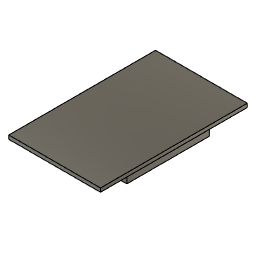
Stack_Up_v2 (Autodesk Fusion 360 archive; units mm, degrees)
design "IO Boards"
Autodesk Fusion 360 part; units mm, degrees
(part 1 of 2)
sketch "Sketch1" plane through (0, 0, 0) normal (0, 0, 1) x (1, 0, 0)
  line L0 (0, 0) -> (40, 0)
  line L1 (40, 0) -> (40, 64)
  line L2 (40, 64) -> (0, 64)
  line L3 (0, 64) -> (0, 0)
  dimension "d1" = 40
  dimension "d2" = 64
  constraint horizontal L0
  constraint vertical L1
  constraint horizontal L2
  constraint vertical L3
  constraint coincident L0.start L3.end
  measures "d1" distance of L0.start L0.end
  measures "d2" distance of L0.start L2.end
extrude "Extrude1" add sketch "Sketch1" along normal blind 1.6
sketch "Sketch4" plane through (0, 0, 0) normal (0, 0, 1) x (1, 0, 0)
  line L0 (0, 0) -> (0, 32) construction
  line L1 (0, 32) -> (40, 32) construction
  line L2 (0, 32) -> (5, 32) construction
  line L3 (40, 32) -> (35, 32) construction
  line L4 (7.5, 50) -> (2.5, 50)
  line L5 (2.5, 50) -> (2.5, 14)
  line L6 (2.5, 14) -> (7.5, 14)
  line L7 (7.5, 14) -> (7.5, 50)
  line L8 (7.5, 50) -> (2.5, 14) construction
  line L9 (2.5, 50) -> (7.5, 14) construction
  line L10 (37.5, 50) -> (32.5, 50)
  line L11 (32.5, 50) -> (32.5, 14)
  line L12 (32.5, 14) -> (37.5, 14)
  line L13 (37.5, 14) -> (37.5, 50)
  line L14 (37.5, 50) -> (32.5, 14) construction
  line L15 (32.5, 50) -> (37.5, 14) construction
  point P0 (5, 32)
  point P1 (35, 32)
  dimension "d23" = 32
  dimension "d24" = 5
  dimension "d25" = 5
  dimension "d26" = 5
  dimension "d27" = 36
  dimension "d28" = 5
  dimension "d29" = 36
  constraint coincident L0.start origin
  constraint vertical L0
  constraint perpendicular L0 L1
  constraint perpendicular L0 L2
  constraint parallel L1 L3
  constraint horizontal L4
  constraint perpendicular L4 L5
  constraint parallel L4 L6
  constraint parallel L5 L7
  constraint coincident L8 P0
  constraint coincident L9 P0
  constraint coincident P0 L2.end
  constraint horizontal L10
  constraint perpendicular L10 L11
  constraint parallel L10 L12
  constraint parallel L11 L13
  constraint coincident L14 P1
  constraint coincident L15 P1
  constraint coincident P1 L3.end
  measures "d23" distance of L0.start L0.end
  measures "d24" distance of L0.end P0
  measures "d25" distance of L1.end P1
  measures "d26" distance of L5.end L6.end
  measures "d27" distance of L4.end L5.end
  measures "d28" distance of L11.end L12.end
  measures "d29" distance of L10.end L11.end
extrude "Extrude6" add sketch "Sketch4" against normal blind 5.08

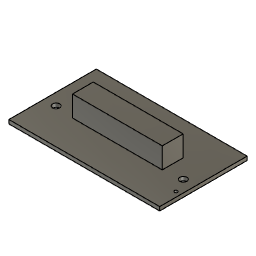
design "Output Board"
Autodesk Fusion 360 part; units mm, degrees
sketch "Sketch1" plane through (0, 0, 0) normal (0, 0, 1) x (1, 0, 0)
  line L0 (0, 0) -> (63.8, 0)
  line L1 (63.8, 0) -> (63.8, 37)
  line L2 (63.8, 37) -> (0, 37)
  line L3 (0, 37) -> (0, 0)
  dimension "d1" = 63.8
  dimension "d2" = 37
  constraint horizontal L0
  constraint vertical L1
  constraint horizontal L2
  constraint vertical L3
  constraint coincident L0.start L3.end
  measures "d1" distance of L0.start L0.end
  measures "d2" distance of L0.start L2.end
extrude "Extrude1" add sketch "Sketch1" along normal blind 1.6
sketch "Sketch2" plane through (0, 0, 1.6) normal (0, 0, 1) x (-1, 0, 0)
  line L0 (0, -37) -> (0, 0)
  line L1 (0, 0) -> (-63.8, 0)
  line L2 (-63.8, 0) -> (-63.8, -37)
  line L3 (-63.8, -37) -> (0, -37)
  line L4 (-50.9, -14) -> (-12.9, -14)
  line L5 (-12.9, -14) -> (-12.9, -22.8)
  line L6 (-12.9, -22.8) -> (-50.9, -22.8)
  line L7 (-50.9, -22.8) -> (-50.9, -14)
  line L8 (-50.9, -14) -> (-12.9, -22.8) construction
  line L9 (-12.9, -14) -> (-50.9, -22.8) construction
  point P0 (-31.9, -18.4)
  dimension "d6" = 38
  dimension "d7" = 8.8
  dimension "d32" = 18.4
  dimension "d33" = 31.9
  constraint horizontal L4
  constraint perpendicular L4 L5
  constraint parallel L4 L6
  constraint parallel L5 L7
  constraint coincident L8 P0
  constraint coincident L9 P0
  measures "d6" distance of L5.end L6.end
  measures "d7" distance of L4.end L5.end
  measures "d32" distance of L1 P0
  measures "d33" distance of L0 P0
extrude "Extrude2" add sketch "Sketch2" along normal blind 8.8 contours L4 L5 L6 L7
sketch "Sketch3" plane through (0, 0, 1.6) normal (0, 0, 1) x (-1, 0, 0)
  line L0 (-50.9, -22.8) -> (-50.9, -14)
  line L1 (-50.9, -14) -> (-12.9, -14)
  line L2 (-12.9, -14) -> (-12.9, -22.8)
  line L3 (-12.9, -22.8) -> (-50.9, -22.8)
  line L4 (0, -37) -> (0, 0)
  line L5 (0, 0) -> (-63.8, 0)
  line L6 (-63.8, 0) -> (-63.8, -37)
  line L7 (-63.8, -37) -> (0, -37)
  circle A0 centre (-58.8, -15) radius 1.5
  circle A1 centre (-5, -15) radius 1.5
  dimension "d10" = 3
  dimension "d12" = 15
  dimension "d13" = 3
  dimension "d19" = 11.6
  dimension "d22" = 5
  dimension "d30" = 58.8
  constraint horizontal A0.centre A1.centre
  measures "d10" diameter of A0
  measures "d12" distance of L5 A0.centre
  measures "d13" diameter of A1
  measures "d22" distance of L4 A1.centre
  measures "d30" distance of L4 A0.centre
extrude "Extrude4" cut sketch "Sketch3" against normal blind 1.6 contours A0 | A1
sketch "Sketch5" plane through (0, 0, 1.6) normal (0, 0, 1) x (-1, 0, 0)
  circle A0 centre (-5, -15) radius 1.5
  circle A1 centre (-58.8, -15) radius 1.5
  line L0 (-50.9, -22.8) -> (-50.9, -14)
  line L1 (-50.9, -14) -> (-12.9, -14)
  line L2 (-12.9, -14) -> (-12.9, -22.8)
  line L3 (-12.9, -22.8) -> (-50.9, -22.8)
  line L4 (0, -37) -> (0, 0)
  line L5 (0, 0) -> (-63.8, 0)
  line L6 (-63.8, 0) -> (-63.8, -37)
  line L7 (-63.8, -37) -> (0, -37)
  circle A2 centre (-61.7, -9) radius 0.655
  dimension "d23" = 1.31
  dimension "d28" = 2.1
  dimension "d29" = 9
  measures "d23" diameter of A2
  measures "d28" distance of L6 A2.centre
  measures "d29" distance of L5 A2.centre
extrude "Extrude5" cut sketch "Sketch5" against normal blind 1.6 contours A2

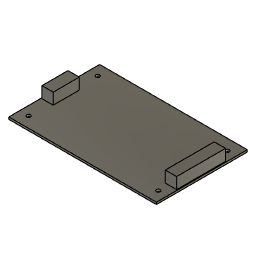
design "Mainboard"
Autodesk Fusion 360 part; units mm, degrees
sketch "Sketch1" plane through (0, 0, 0) normal (0, 0, 1) x (1, 0, 0)
  line L0 (0, 0) -> (115, 0)
  line L1 (115, 0) -> (115, 70.8)
  line L2 (115, 70.8) -> (0, 70.8)
  line L3 (0, 70.8) -> (0, 0)
  line L4 (0, 0) -> (0, 2)
  line L5 (0, 2) -> (115, 2)
  line L6 (0, 70.8) -> (0, 68.8)
  line L7 (0, 68.8) -> (115, 68.8)
  dimension "d1" = 70.8
  dimension "d2" = 115
  dimension "d5" = 2
  dimension "d6" = 2
  constraint horizontal L0
  constraint vertical L1
  constraint horizontal L2
  constraint vertical L3
  constraint coincident L0.start L3.end
  constraint perpendicular L0 L4
  constraint coincident L1 L5.end
  constraint perpendicular L1 L5
  constraint perpendicular L2 L6
  constraint coincident L1 L7.end
  constraint perpendicular L1 L7
  measures "d1" distance of L0.start L2.end
  measures "d2" distance of L0.start L0.end
  measures "d5" distance of L0.start L4.end
  measures "d6" distance of L2.end L6.end
extrude "Extrude1" add sketch "Sketch1" along normal blind 1.6
sketch "Sketch2" plane through (0, 0, 1.6) normal (0, 0, 1) x (-1, 0, 0)
  line L0 (0, -70.8) -> (0, 0)
  line L1 (0, 0) -> (-115, 0)
  line L2 (-115, 0) -> (-115, -70.8)
  line L3 (-115, -70.8) -> (0, -70.8)
  line L4 (0, 0) -> (0, -70.8) construction
  line L5 (0, -35.4) -> (-5, -35.4)
  line L6 (-9.4, -25.25) -> (-0.6, -25.25)
  line L7 (-0.6, -25.25) -> (-0.6, -45.55)
  line L8 (-0.6, -45.55) -> (-9.4, -45.55)
  line L9 (-9.4, -45.55) -> (-9.4, -25.25)
  line L10 (-9.4, -25.25) -> (-0.6, -45.55) construction
  line L11 (-0.6, -25.25) -> (-9.4, -45.55) construction
  line L12 (0, -35.4) -> (-110, -35.4) construction
  line L13 (-114.4, -54.44) -> (-105.6, -54.44)
  line L14 (-105.6, -54.44) -> (-105.6, -16.36)
  line L15 (-105.6, -16.36) -> (-114.4, -16.36)
  line L16 (-114.4, -16.36) -> (-114.4, -54.44)
  line L17 (-114.4, -54.44) -> (-105.6, -16.36) construction
  line L18 (-105.6, -54.44) -> (-114.4, -16.36) construction
  point P0 (-5, -35.4)
  point P1 (-110, -35.4)
  dimension "d7" = 5
  dimension "d8" = 8.8
  dimension "d9" = 20.3
  dimension "d10" = 110
  dimension "d11" = 8.8
  dimension "d12" = 38.08
  constraint coincident L0.end L1.start
  constraint coincident L0.start L3.end
  constraint midpoint L4 L5.start
  constraint perpendicular L0 L5
  constraint horizontal L6
  constraint perpendicular L6 L7
  constraint parallel L6 L8
  constraint parallel L7 L9
  constraint coincident L10 P0
  constraint coincident L11 P0
  constraint coincident P0 L5.end
  constraint perpendicular L2 L12
  constraint horizontal L13
  constraint perpendicular L13 L14
  constraint parallel L13 L15
  constraint parallel L14 L16
  constraint coincident L17 P1
  constraint coincident L18 P1
  constraint coincident P1 L12.end
  measures "d7" distance of L5.start P0
  measures "d8" distance of L7.end L8.end
  measures "d9" distance of L6.end L7.end
  measures "d10" distance of L5.start P1
  measures "d11" distance of L14.end L15.end
  measures "d12" distance of L13.end L14.end
extrude "Extrude2" add sketch "Sketch2" along normal blind 8.8 contours L6 L7 L8 L9 | L13 L14 L15 L16
sketch "Sketch3" plane through (0, 0, 1.6) normal (0, 0, 1) x (-1, 0, 0)
  line L0 (-9.4, -45.55) -> (-9.4, -25.25)
  line L1 (-9.4, -25.25) -> (-0.6, -25.25)
  line L2 (-0.6, -25.25) -> (-0.6, -45.55)
  line L3 (-0.6, -45.55) -> (-9.4, -45.55)
  line L4 (-114.4, -16.36) -> (-105.6, -16.36)
  line L5 (-105.6, -16.36) -> (-105.6, -54.44)
  line L6 (-105.6, -54.44) -> (-114.4, -54.44)
  line L7 (-114.4, -54.44) -> (-114.4, -16.36)
  line L8 (0, -70.8) -> (0, 0)
  line L9 (0, 0) -> (-115, 0)
  line L10 (-115, 0) -> (-115, -70.8)
  line L11 (-115, -70.8) -> (0, -70.8)
  circle A0 centre (-7, -8.5) radius 1.5
  circle A1 centre (-7, -62.3) radius 1.5
  circle A2 centre (-108, -62.3) radius 1.5
  circle A3 centre (-108, -8.5) radius 1.5
  dimension "d15" = 3
  dimension "d16" = 7
  dimension "d17" = 8.5
  dimension "d18" = 3
  dimension "d19" = 62.3
  dimension "d20" = 7
  dimension "d21" = 3
  dimension "d22" = 108
  dimension "d23" = 62.3
  dimension "d24" = 3
  dimension "d25" = 8.5
  dimension "d26" = 108
  measures "d15" diameter of A0
  measures "d16" distance of L8 A0.centre
  measures "d17" distance of L9 A0.centre
  measures "d18" diameter of A1
  measures "d19" distance of L9 A1.centre
  measures "d20" distance of L8 A1.centre
  measures "d21" diameter of A2
  measures "d22" horizontal distance of L8.end A2.centre
  measures "d23" vertical distance of L8.end A2.centre
  measures "d24" diameter of A3
  measures "d25" vertical distance of L8.end A3.centre
  measures "d26" horizontal distance of L8.end A3.centre
extrude "Extrude3" cut sketch "Sketch3" against normal blind 1.6 contours A0 | A1 | A2 | A3

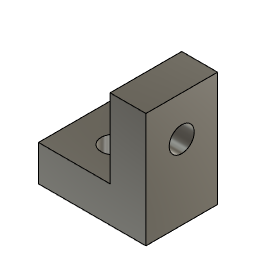
design "Output_Bot_Stand"
Autodesk Fusion 360 part; units mm, degrees
sketch "Sketch1" plane through (0, 0, 0) normal (0, 0, 1) x (1, 0, 0)
  line L0 (0, 0) -> (15, 0)
  line L1 (15, 0) -> (15, 10)
  line L2 (15, 10) -> (0, 10)
  line L3 (0, 10) -> (0, 0)
  line L4 (15, 5) -> (5.5, 5)
  circle A0 centre (5.5, 5) radius 1.75
  dimension "d1" = 15
  dimension "d2" = 10
  dimension "d27" = 9.5
  dimension "d28" = 3.5
  constraint horizontal L0
  constraint vertical L1
  constraint horizontal L2
  constraint vertical L3
  constraint coincident L0.start L3.end
  constraint midpoint L1 L4.start
  constraint perpendicular L1 L4
  constraint coincident L4.end A0.centre
  measures "d1" distance of L0.start L0.end
  measures "d2" distance of L0.start L2.end
  measures "d27" distance of L4.start L4.end
  measures "d28" diameter of A0
extrude "Extrude1" add sketch "Sketch1" along normal blind 5 contours L0 L1 L2 L3 | A0
extrude "Extrude4" cut sketch "Sketch1" along normal blind 5 contours A0
sketch "Sketch5" plane through (0, 0, 0) normal (0, 0, -1) x (1, 0, 0)
  circle A0 centre (5.5, -5) radius 1.75
  line L0 (0, 0) -> (0, -10)
  line L1 (0, -10) -> (15, -10)
  line L2 (15, -10) -> (15, 0)
  line L3 (15, 0) -> (0, 0)
  line L4 (15, 0) -> (10, 0)
  line L5 (10, 0) -> (10, -10)
  line L6 (10, -10) -> (15, -10)
  line L7 (15, -10) -> (15, 0)
  dimension "d31" = 5
  dimension "d32" = 10
  constraint horizontal L4
  constraint vertical L5
  constraint horizontal L6
  constraint vertical L7
  constraint coincident L2.end L3.start
  measures "d31" distance of L2.end L4.end
  measures "d32" distance of L2.end L1.end
extrude "Extrude5" add sketch "Sketch5" against normal blind 16 contours L1 L2 L3 L4 L5 L6 L7
sketch "Sketch6" plane through (15, 0, 0) normal (1, 0, 0) x (0, 1, 0)
  line L0 (0, 0) -> (10, 0)
  line L1 (10, 0) -> (10, 16)
  line L2 (10, 16) -> (0, 16)
  line L3 (0, 16) -> (0, 0)
  line L4 (5, 0) -> (5, 10.4)
  circle A0 centre (5, 10.4) radius 1.75
  dimension "d35" = 10.4
  dimension "d36" = 3.5
  constraint midpoint L0 L4.start
  constraint perpendicular L0 L4
  constraint coincident L4.end A0.centre
  measures "d35" distance of L4.start L4.end
  measures "d36" diameter of A0
extrude "Extrude6" cut sketch "Sketch6" against normal blind 5 contours A0

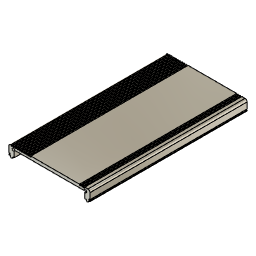
design "Top Half"
Autodesk Fusion 360 part; units mm, degrees
sketch "Sketch1" plane through (0, 0, 0) normal (0, 1, 0) x (1, 0, 0)
  line L0 (74.3, 0) -> (75.5, 0)
  line L1 (73.6, -1.4134) -> (74.3, 0)
  line L2 (77.4, -36.6134) -> (76.2, -36.6134)
  arc A0 (75.4, -10.8) -> (77.4, -8.8) centre (75.4, -8.8) ccw
  line L3 (0, -1.4134) -> (1.2, -1.4134)
  line L4 (72.4, -1.4134) -> (73.6, -1.4134)
  line L5 (77.4, -1.4134) -> (76.2, -1.4134)
  line L6 (75.5, 0) -> (76.2, -1.4134)
  line L7 (72.4, -36.6134) -> (73.6, -36.6134)
  line L8 (3.1, 0) -> (3.8, -1.4134)
  arc A1 (71.75, -7.8) -> (72.4, -6.7034) centre (73, -7.8) ccw
  line L9 (5.5312, -7.8) -> (71.75, -7.8)
  line L10 (1.9, 0) -> (3.1, 0)
  line L11 (1.2, -1.4134) -> (1.9, 0)
  line L12 (5, -1.4134) -> (3.8, -1.4134)
  arc A2 (0, -8.8) -> (2, -10.8) centre (2, -8.8) ccw
  arc A3 (5, -6.8511) -> (5.5312, -7.8) centre (4.2835, -7.8754) ccw
  line L13 (75.4, -10.8) -> (2, -10.8)
  line L14 (75.5, -35.2) -> (76.2, -36.6134)
  line L15 (73.6, -36.6134) -> (74.3, -35.2)
  line L16 (74.3, -35.2) -> (75.5, -35.2)
  line L17 (5, -6.8511) -> (5, -1.4134)
  line L18 (0, -8.8) -> (0, -1.4134)
  line L19 (72.4, -6.7034) -> (72.4, -1.4134)
  line L20 (77.4, -8.8) -> (77.4, -1.4134)
  point P0 (77.4, -10.8)
  point P1 (0, -10.8)
  dimension "d2" = 77.4
  dimension "d3" = 2
  dimension "d4" = 2
  dimension "d9" = 3
  dimension "d17" = 2.5
  dimension "d18" = 2.5
  dimension "d21" = 67.4
  dimension "d23" = 1.2
  dimension "d24" = 1.2
  dimension "d25" = 1.2
  dimension "d26" = 1.2
  dimension "d27" = 1.2
  dimension "d28" = 1.2
  dimension "d29" = 1.2
  dimension "d30" = 1.2
  dimension "d31" = 1.2
  constraint horizontal L13
  constraint coincident P1 L13
  constraint tangent A2 L13
  constraint coincident P0 L13
  constraint tangent A0 L13
  constraint horizontal L9
  constraint collinear L4 L5
  constraint collinear L2 L7
  constraint collinear L3 L12
  constraint perpendicular L12 L17
  constraint tangent A2 L18
  constraint perpendicular L4 L19
  constraint tangent A0 L20
  constraint coincident origin L10
  measures "d2" distance of P0 P1
  measures "d3" radius of A2
  measures "d4" radius of A0
  measures "d9" distance of L9 L13
  measures "d17" diameter of A3
  measures "d18" diameter of A1
  measures "d21" horizontal distance of A3.start A1.end
  measures "d23" distance of L1.start L4.start
  measures "d24" distance of L5.start L5.end
  measures "d25" distance of L0.start L0.end
  measures "d26" distance of L7.end L7.start
  measures "d27" distance of L2.start L2.end
  measures "d28" distance of L15.end L14.start
  measures "d29" distance of L3.end L3.start
  measures "d30" distance of L12.start L8.end
  measures "d31" distance of L8.start L10.start
extrude "Extrude1" add sketch "Sketch1" along normal blind 150
sketch "Sketch2" plane through (0, 0, 10.8) normal (0, 0, 1) x (-1, 0, 0)
  line L0 (-2, 0) -> (-75.4, 0)
  line L1 (-75.4, 0) -> (-75.4, -150)
  line L2 (-75.4, -150) -> (-2, -150)
  line L3 (-2, -150) -> (-2, 0)
  line L4 (-19, 0) -> (-18, 0)
  line L5 (-20, 0) -> (-20, -150)
  line L6 (-13, 0) -> (-12, 0)
  line L7 (-5, -150) -> (-5, 0)
  line L8 (-2, 0) -> (-2, -150)
  line L9 (-10, 0) -> (-10, -150)
  line L10 (-15, 0) -> (-14, 0)
  line L11 (-15, -150) -> (-15, 0)
  line L12 (-11, -150) -> (-11, 0)
  line L13 (-4, 0) -> (-4, -150)
  line L14 (-7, 0) -> (-6, 0)
  line L15 (-19, -150) -> (-19, 0)
  line L16 (-3, -150) -> (-3, 0)
  line L17 (-8, 0) -> (-8, -150)
  line L18 (-16, 0) -> (-16, -150)
  line L19 (-11, 0) -> (-10, 0)
  line L20 (-18, -150) -> (-19, -150)
  line L21 (-2, -150) -> (-3, -150)
  line L22 (-6, 0) -> (-6, -150)
  line L23 (-21, 0) -> (-20, 0)
  line L24 (-13, -150) -> (-13, 0)
  line L25 (-17, -150) -> (-17, 0)
  line L26 (-5, 0) -> (-4, 0)
  line L27 (-14, 0) -> (-14, -150)
  line L28 (-12, 0) -> (-12, -150)
  line L29 (-9, -150) -> (-9, 0)
  line L30 (-3, 0) -> (-2, 0)
  line L31 (-75.4, -150) -> (-2, -150)
  line L32 (-68.4, -150) -> (-67.4, -150)
  line L33 (-9, 0) -> (-8, 0)
  line L34 (-7, -150) -> (-7, 0)
  line L35 (-75.4, 0) -> (-75.4, -150)
  line L36 (-2, -150) -> (-2, 0)
  line L37 (-69.4, 0) -> (-70.4, 0)
  line L38 (-68.4, 0) -> (-68.4, -150)
  line L39 (-2, 0) -> (-75.4, 0)
  line L40 (-69.4, -150) -> (-69.4, 0)
  line L41 (-72.4, 0) -> (-72.4, -150)
  line L42 (-71.4, 0) -> (-72.4, 0)
  line L43 (-4, -150) -> (-5, -150)
  line L44 (-67.4, -150) -> (-67.4, 0)
  line L45 (-10, -150) -> (-11, -150)
  line L46 (-14, -150) -> (-15, -150)
  line L47 (-16, -150) -> (-17, -150)
  line L48 (-12, -150) -> (-13, -150)
  line L49 (-18, 0) -> (-18, -150)
  line L50 (-70.4, 0) -> (-70.4, -150)
  line L51 (-21, -150) -> (-21, 0)
  line L52 (-8, -150) -> (-9, -150)
  line L53 (-6, -150) -> (-7, -150)
  line L54 (-70.4, -150) -> (-69.4, -150)
  line L55 (-17, 0) -> (-16, 0)
  line L56 (-71.4, -150) -> (-71.4, 0)
  line L57 (-67.4, 0) -> (-68.4, 0)
  line L58 (-20, -150) -> (-21, -150)
  line L59 (-72.4, -150) -> (-71.4, -150)
  dimension "d38" = 1
  dimension "d39" = 150
  dimension "d40" = 1
  dimension "d41" = 150
  dimension "d42" = 1
  dimension "d43" = 150
  dimension "d44" = 1
  dimension "d45" = 150
  dimension "d46" = 1
  dimension "d47" = 150
  dimension "d48" = 1
  dimension "d49" = 150
  dimension "d50" = 1
  dimension "d51" = 150
  dimension "d52" = 1
  dimension "d53" = 150
  dimension "d54" = 1
  dimension "d55" = 150
  dimension "d56" = 1
  dimension "d57" = 150
  dimension "d58" = 1
  dimension "d59" = 1
  dimension "d60" = 1
  dimension "d61" = 1
  dimension "d62" = 1
  dimension "d63" = 1
  dimension "d64" = 1
  dimension "d65" = 1
  dimension "d66" = 1
  dimension "d67" = 1
  dimension "d68" = 150
  dimension "d69" = 3
  dimension "d70" = 1
  dimension "d71" = 150
  dimension "d72" = 1
  dimension "d73" = 150
  dimension "d74" = 1
  dimension "d75" = 1
  constraint horizontal L21
  constraint vertical L16
  constraint horizontal L30
  constraint vertical L8
  constraint coincident L2.end L3.start
  constraint horizontal L43
  constraint vertical L7
  constraint horizontal L26
  constraint vertical L13
  constraint coincident L13.end L31
  constraint horizontal L53
  constraint vertical L34
  constraint horizontal L14
  constraint vertical L22
  constraint coincident L22.end L31
  constraint horizontal L52
  constraint vertical L29
  constraint horizontal L33
  constraint vertical L17
  constraint coincident L17.end L31
  constraint horizontal L45
  constraint vertical L12
  constraint horizontal L19
  constraint vertical L9
  constraint coincident L9.end L31
  constraint horizontal L48
  constraint vertical L24
  constraint horizontal L6
  constraint vertical L28
  constraint coincident L28.end L31
  constraint horizontal L46
  constraint vertical L11
  constraint horizontal L10
  constraint vertical L27
  constraint coincident L27.end L31
  constraint horizontal L47
  constraint vertical L25
  constraint horizontal L55
  constraint vertical L18
  constraint coincident L18.end L31
  constraint horizontal L20
  constraint vertical L15
  constraint horizontal L4
  constraint vertical L49
  constraint coincident L20.start L31
  constraint horizontal L58
  constraint vertical L51
  constraint horizontal L23
  constraint vertical L5
  constraint coincident L5.end L31
  constraint horizontal L59
  constraint vertical L56
  constraint horizontal L42
  constraint vertical L41
  constraint coincident L41.end L31
  constraint horizontal L54
  constraint vertical L40
  constraint horizontal L37
  constraint vertical L50
  constraint coincident L50.end L31
  constraint horizontal L32
  constraint vertical L44
  constraint horizontal L57
  constraint vertical L38
  constraint coincident L32.start L31
  measures "d38" distance of L2.end L16.start
  measures "d39" distance of L2.end L0.start
  measures "d40" distance of L13.end L7.start
  measures "d41" distance of L13.end L13.start
  measures "d42" distance of L22.end L34.start
  measures "d43" distance of L22.end L14.end
  measures "d44" distance of L29.start L17.end
  measures "d45" distance of L17.start L17.end
  measures "d46" distance of L12.start L9.end
  measures "d47" distance of L9.start L9.end
  measures "d48" distance of L28.end L24.start
  measures "d49" distance of L28.end L6.end
  measures "d50" distance of L11.start L27.end
  measures "d51" distance of L27.end L10.end
  measures "d52" distance of L18.end L25.start
  measures "d53" distance of L18.end L18.start
  measures "d54" distance of L20.start L15.start
  measures "d55" distance of L20.start L4.end
  measures "d56" distance of L51.start L5.end
  measures "d57" distance of L5.end L5.start
  measures "d58" distance of L13 L16
  measures "d59" distance of L7 L22
  measures "d60" distance of L17 L34
  measures "d61" distance of L9 L29
  measures "d62" distance of L12 L28
  measures "d63" distance of L24 L27
  measures "d64" distance of L11 L18
  measures "d65" distance of L25 L49
  measures "d66" distance of L5 L15
  measures "d67" distance of L41.end L56.start
  measures "d68" distance of L41.end L41.start
  measures "d69" distance of L35 L41
  measures "d70" distance of L50.end L40.start
  measures "d71" distance of L50.end L37.end
  measures "d72" distance of L32.start L32.end
  measures "d73" distance of L32.start L38.start
  measures "d74" distance of L38 L40
  measures "d75" distance of L50 L56
extrude "Extrude2" cut sketch "Sketch2" against normal blind 1 contours L0 L2 L3 L8 L16 L21 L30 L31 L36 L39 | L0 L2 L7 L13 L26 L31 L39 L43 | L0 L2 L14 L22 L31 L34 L39 L53 | L0 L2 L17 L29 L31 L33 L39 L52 | L0 L2 L9 L12 L19 L31 L39 L45 | L0 L2 L6 L24 L28 L31 L39 L48 | L0 L2 L10 L11 L27 L31 L39 L46 | L0 L2 L18 L25 L31 L39 L47 L55 | L0 L2 L4 L15 L20 L31 L39 L49 | L0 L2 L5 L23 L31 L39 L51 L58 | L0 L2 L31 L32 L38 L39 L44 L57 | L0 L2 L31 L37 L39 L40 L50 L54 | L0 L2 L31 L39 L41 L42 L56 L59
sketch "Sketch3" plane through (77.4, 0, 0) normal (1, 0, 0) x (0, 1, 0)
  line L0 (0, 8.8) -> (0, 1.4134)
  line L1 (0, 1.4134) -> (150, 1.4134)
  line L2 (150, 1.4134) -> (150, 8.8)
  line L3 (150, 8.8) -> (0, 8.8)
  line L4 (150, 3) -> (150, 2)
  line L5 (150, -1) -> (150, -2)
  line L6 (150, -31) -> (150, -30)
  line L7 (150, -27) -> (150, -26)
  line L8 (150, -7) -> (150, -8)
  line L9 (150, -3) -> (150, -4)
  line L10 (150, 1) -> (150, 0)
  line L11 (0, -27) -> (150, -27)
  line L12 (150, -8) -> (0, -8)
  line L13 (0, 1) -> (150, 1)
  line L14 (150, -24) -> (150, -25)
  line L15 (150, -5) -> (150, -6)
  line L16 (150, -29) -> (150, -28)
  line L17 (0, 2) -> (0, 3)
  line L18 (150, -2) -> (0, -2)
  line L19 (150, 9) -> (0, 9)
  line L20 (0, 0) -> (0, 1)
  line L21 (0, -31) -> (150, -31)
  line L22 (150, -25) -> (0, -25)
  line L23 (0, -24) -> (150, -24)
  line L24 (150, -30) -> (0, -30)
  line L25 (0, -30) -> (0, -31)
  line L26 (150, -33) -> (150, 9)
  line L27 (0, -5) -> (150, -5)
  line L28 (0, -7) -> (150, -7)
  line L29 (0, -33) -> (150, -33)
  line L30 (0, 9) -> (0, -33)
  line L31 (0, -29) -> (150, -29)
  line L32 (0, -3) -> (150, -3)
  line L33 (0, -28) -> (0, -29)
  line L34 (150, 0) -> (0, 0)
  line L35 (0, -25) -> (0, -24)
  line L36 (150, -26) -> (0, -26)
  line L37 (0, -1) -> (150, -1)
  line L38 (0, -4) -> (0, -3)
  line L39 (0, -2) -> (0, -1)
  line L40 (0, -26) -> (0, -27)
  line L41 (0, -8) -> (0, -7)
  line L42 (0, 3) -> (150, 3)
  line L43 (0, -6) -> (0, -5)
  line L44 (150, 2) -> (0, 2)
  line L45 (150, -4) -> (0, -4)
  line L46 (150, -6) -> (0, -6)
  line L47 (150, -28) -> (0, -28)
  point P0 (0, -35)
  dimension "d111" = 150
  dimension "d112" = 1
  dimension "d113" = 150
  dimension "d114" = 1
  dimension "d115" = 150
  dimension "d116" = 1
  dimension "d117" = 150
  dimension "d118" = 1
  dimension "d119" = 150
  dimension "d120" = 1
  dimension "d121" = 150
  dimension "d122" = 1
  dimension "d123" = 150
  dimension "d124" = 1
  dimension "d125" = 150
  dimension "d126" = 1
  dimension "d127" = 150
  dimension "d128" = 1
  dimension "d129" = 150
  dimension "d130" = 1
  constraint horizontal L42
  constraint vertical L4
  constraint horizontal L44
  constraint vertical L17
  constraint coincident L17.end L30
  constraint horizontal L13
  constraint vertical L10
  constraint horizontal L34
  constraint vertical L20
  constraint coincident L13.start L30
  constraint horizontal L37
  constraint vertical L5
  constraint horizontal L18
  constraint vertical L39
  constraint coincident L37.start L30
  constraint horizontal L32
  constraint vertical L9
  constraint horizontal L45
  constraint vertical L38
  constraint coincident L32.start L30
  constraint horizontal L27
  constraint vertical L15
  constraint horizontal L46
  constraint vertical L43
  constraint coincident L27.start L30
  constraint horizontal L28
  constraint vertical L8
  constraint horizontal L12
  constraint vertical L41
  constraint coincident L28.start L30
  constraint horizontal L21
  constraint vertical L6
  constraint horizontal L24
  constraint vertical L25
  constraint coincident L21.start L30
  constraint horizontal L31
  constraint vertical L16
  constraint horizontal L47
  constraint vertical L33
  constraint coincident L31.start L30
  constraint horizontal L11
  constraint vertical L7
  constraint horizontal L36
  constraint vertical L40
  constraint coincident L11.start L30
  constraint horizontal L23
  constraint vertical L14
  constraint horizontal L22
  constraint vertical L35
  constraint coincident L23.start L30
  measures "d111" distance of L4.start L17.end
  measures "d112" distance of L17.start L17.end
  measures "d113" distance of L10.start L13.start
  measures "d114" distance of L13.start L20.start
  measures "d115" distance of L5.start L37.start
  measures "d116" distance of L18.end L37.start
  measures "d117" distance of L32.start L9.start
  measures "d118" distance of L38.start L32.start
  measures "d119" distance of L27.start L15.start
  measures "d120" distance of L27.start L43.start
  measures "d121" distance of L28.start L8.start
  measures "d122" distance of L28.start L12.end
  measures "d123" distance of L21.start L6.start
  measures "d124" distance of L24.end L21.start
  measures "d125" distance of L31.start L16.start
  measures "d126" distance of L33.start L31.start
  measures "d127" distance of L7.start L11.start
  measures "d128" distance of L11.start L36.end
  measures "d129" distance of L23.start L14.start
  measures "d130" distance of L23.start L22.end
extrude "Extrude3" cut sketch "Sketch3" against normal blind 1 contours L0 L2 L4 L17 L26 L30 L42 L44
sketch "Sketch4" plane through (0, 0, 0) normal (-1, 0, 0) x (0, -1, 0)
  line L0 (0, 1.4134) -> (0, 8.8)
  line L1 (0, 8.8) -> (-150, 8.8)
  line L2 (-150, 8.8) -> (-150, 1.4134)
  line L3 (-150, 1.4134) -> (0, 1.4134)
  line L4 (0, -33) -> (0, 1.6134)
  line L5 (-150, -33) -> (0, -33)
  line L6 (0, 1.6134) -> (-150, 1.6134)
  line L7 (-150, 1) -> (0, 1)
  line L8 (0, -26) -> (-150, -26)
  line L9 (-150, -28) -> (-150, -29)
  line L10 (-150, -30) -> (-150, -31)
  line L11 (-150, -5) -> (0, -5)
  line L12 (-150, -1) -> (0, -1)
  line L13 (-150, -29) -> (0, -29)
  line L14 (-150, -8) -> (-150, -7)
  line L15 (-150, 2) -> (-150, 3)
  line L16 (0, -2) -> (-150, -2)
  line L17 (0, -30) -> (-150, -30)
  line L18 (0, 2) -> (-150, 2)
  line L19 (0, -4) -> (-150, -4)
  line L20 (0, -1) -> (0, -2)
  line L21 (-150, -33) -> (0, -33)
  line L22 (-150, -25) -> (-150, -24)
  line L23 (0, -27) -> (0, -26)
  line L24 (-150, 0) -> (-150, 1)
  line L25 (0, -29) -> (0, -28)
  line L26 (0, -5) -> (0, -6)
  line L27 (0, -31) -> (0, -30)
  line L28 (-150, -4) -> (-150, -3)
  line L29 (-150, 9) -> (-150, -33)
  line L30 (-150, -26) -> (-150, -27)
  line L31 (0, -6) -> (-150, -6)
  line L32 (0, -3) -> (0, -4)
  line L33 (0, -7) -> (0, -8)
  line L34 (-150, -24) -> (0, -24)
  line L35 (-150, 1.6134) -> (-150, -33)
  line L36 (-150, -7) -> (0, -7)
  line L37 (-150, -31) -> (0, -31)
  line L38 (0, -28) -> (-150, -28)
  line L39 (-150, 3) -> (0, 3)
  line L40 (-150, -27) -> (0, -27)
  line L41 (0, 1) -> (0, 0)
  line L42 (0, -24) -> (0, -25)
  line L43 (0, 0) -> (-150, 0)
  line L44 (0, -33) -> (0, 9)
  line L45 (-150, -3) -> (0, -3)
  line L46 (-150, -6) -> (-150, -5)
  line L47 (0, -25) -> (-150, -25)
  line L48 (0, 9) -> (-150, 9)
  line L49 (0, -8) -> (-150, -8)
  line L50 (-150, -2) -> (-150, -1)
  line L51 (0, 3) -> (0, 2)
  point P0 (-150, -35)
  point P1 (0, -35)
  dimension "d100" = 150
  dimension "d101" = 1
  dimension "d102" = 150
  dimension "d103" = 1
  dimension "d104" = 150
  dimension "d105" = 1
  dimension "d106" = 150
  dimension "d107" = 1
  dimension "d108" = 150
  dimension "d109" = 1
  dimension "d110" = 150
  dimension "d131" = 1
  dimension "d132" = 150
  dimension "d133" = 1
  dimension "d134" = 150
  dimension "d135" = 1
  dimension "d136" = 150
  dimension "d137" = 1
  dimension "d138" = 150
  dimension "d139" = 1
  constraint horizontal L39
  constraint vertical L51
  constraint horizontal L18
  constraint vertical L15
  constraint coincident L15.end L29
  constraint horizontal L7
  constraint vertical L41
  constraint horizontal L43
  constraint vertical L24
  constraint coincident L7.start L29
  constraint horizontal L12
  constraint vertical L20
  constraint horizontal L16
  constraint vertical L50
  constraint coincident L12.start L29
  constraint horizontal L45
  constraint vertical L32
  constraint horizontal L19
  constraint vertical L28
  constraint coincident L28.end L29
  constraint horizontal L11
  constraint vertical L26
  constraint horizontal L31
  constraint vertical L46
  constraint coincident L11.start L29
  constraint horizontal L36
  constraint vertical L33
  constraint horizontal L49
  constraint vertical L14
  constraint coincident L14.end L29
  constraint horizontal L37
  constraint vertical L27
  constraint horizontal L17
  constraint vertical L10
  constraint coincident L10.end L29
  constraint horizontal L13
  constraint vertical L25
  constraint horizontal L38
  constraint vertical L9
  constraint coincident L9.end L29
  constraint horizontal L40
  constraint vertical L23
  constraint horizontal L8
  constraint vertical L30
  constraint coincident L30.end L29
  constraint horizontal L34
  constraint vertical L42
  constraint horizontal L47
  constraint vertical L22
  constraint coincident L22.end L29
  measures "d100" distance of L15.end L39.end
  measures "d101" distance of L15.start L15.end
  measures "d102" distance of L7.start L7.end
  measures "d103" distance of L24.start L7.start
  measures "d104" distance of L12.end L12.start
  measures "d105" distance of L16.end L12.start
  measures "d106" distance of L28.end L32.start
  measures "d107" distance of L19.end L28.end
  measures "d108" distance of L11.end L11.start
  measures "d109" distance of L11.start L31.end
  measures "d110" distance of L14.end L33.start
  measures "d131" distance of L14.start L14.end
  measures "d132" distance of L10.end L27.start
  measures "d133" distance of L10.start L10.end
  measures "d134" distance of L13.end L9.end
  measures "d135" distance of L9.start L9.end
  measures "d136" distance of L23.start L30.end
  measures "d137" distance of L8.end L30.end
  measures "d138" distance of L34.end L22.end
  measures "d139" distance of L22.start L22.end
extrude "Extrude4" cut sketch "Sketch4" against normal blind 1 contours L0 L2 L15 L18 L29 L39 L44 L51

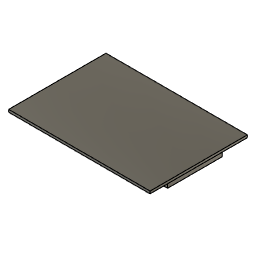
design "DO_Board"
Autodesk Fusion 360 part; units mm, degrees
sketch "Sketch1" plane through (0, 0, 0) normal (0, 0, 1) x (1, 0, 0)
  line L0 (0, 0) -> (93, 0)
  line L1 (93, 0) -> (93, 64)
  line L2 (93, 64) -> (0, 64)
  line L3 (0, 64) -> (0, 0)
  dimension "d1" = 93
  dimension "d2" = 64
  constraint horizontal L0
  constraint vertical L1
  constraint horizontal L2
  constraint vertical L3
  constraint coincident L0.start L3.end
  measures "d1" distance of L0.start L0.end
  measures "d2" distance of L0.start L2.end
extrude "Extrude1" add sketch "Sketch1" along normal blind 1.6
sketch "Sketch2" plane through (0, 0, 0) normal (0, 0, -1) x (1, 0, 0)
  line L0 (0, 0) -> (0, -64)
  line L1 (0, -64) -> (93, -64)
  line L2 (93, -64) -> (93, 0)
  line L3 (93, 0) -> (0, 0)
  line L4 (93, 0) -> (93, -32) construction
  line L5 (93, -32) -> (88, -32) construction
  line L6 (90.5, -50) -> (85.5, -50)
  line L7 (85.5, -50) -> (85.5, -14)
  line L8 (85.5, -14) -> (90.5, -14)
  line L9 (90.5, -14) -> (90.5, -50)
  line L10 (90.5, -50) -> (85.5, -14) construction
  line L11 (85.5, -50) -> (90.5, -14) construction
  line L12 (88, -32) -> (58, -32) construction
  line L13 (60.5, -50) -> (55.5, -50)
  line L14 (55.5, -50) -> (55.5, -14)
  line L15 (55.5, -14) -> (60.5, -14)
  line L16 (60.5, -14) -> (60.5, -50)
  line L17 (60.5, -50) -> (55.5, -14) construction
  line L18 (55.5, -50) -> (60.5, -14) construction
  point P0 (88, -32)
  point P1 (58, -32)
  dimension "d5" = 32
  dimension "d6" = 5
  dimension "d7" = 5
  dimension "d8" = 36
  dimension "d11" = 30
  dimension "d12" = 5
  dimension "d13" = 36
  constraint coincident L2.end L3.start
  constraint perpendicular L3 L4
  constraint perpendicular L4 L5
  constraint horizontal L6
  constraint perpendicular L6 L7
  constraint parallel L6 L8
  constraint parallel L7 L9
  constraint coincident L10 P0
  constraint coincident L11 P0
  constraint coincident P0 L5.end
  constraint perpendicular L7 L12
  constraint horizontal L13
  constraint perpendicular L13 L14
  constraint parallel L13 L15
  constraint parallel L14 L16
  constraint coincident L17 P1
  constraint coincident L18 P1
  constraint coincident P1 L12.end
  measures "d5" distance of L2.end L4.end
  measures "d6" distance of L4.end P0
  measures "d7" distance of L7.end L8.end
  measures "d8" distance of L6.end L7.end
  measures "d11" distance of P0 P1
  measures "d12" distance of L14.end L15.end
  measures "d13" distance of L13.end L14.end
extrude "Extrude2" add sketch "Sketch2" along normal blind 5.08 contours L6 L7 L8 L9 | L13 L14 L15 L16

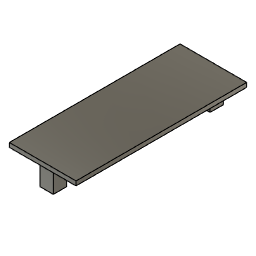
design "Powerboards"
Autodesk Fusion 360 part; units mm, degrees
sketch "Sketch1" plane through (0, 0, 0) normal (0, 0, 1) x (1, 0, 0)
  line L0 (25, 0) -> (25, 64)
  line L1 (0, 64) -> (0, 0)
  line L2 (17.77, 57.5) -> (9.77, 57.5)
  line L3 (9.77, 57.5) -> (9.77, 62.5)
  line L4 (9.77, 62.5) -> (17.77, 62.5)
  line L5 (17.77, 62.5) -> (17.77, 57.5)
  line L6 (17.77, 57.5) -> (9.77, 62.5) construction
  line L7 (9.77, 57.5) -> (17.77, 62.5) construction
  line L8 (15, 6.5) -> (10, 6.5)
  line L9 (10, 6.5) -> (10, 1.5)
  line L10 (10, 1.5) -> (15, 1.5)
  line L11 (15, 1.5) -> (15, 6.5)
  line L12 (15, 6.5) -> (10, 1.5) construction
  line L13 (10, 6.5) -> (15, 1.5) construction
  line L14 (0, 0) -> (12.5, 0) construction
  line L15 (12.5, 0) -> (12.5, 4) construction
  line L16 (0, 0) -> (25, 0)
  line L17 (13.77, 60) -> (13.77, 0) construction
  line L18 (13.77, 60) -> (0, 60) construction
  line L19 (0, 64) -> (25, 64)
  point P0 (13.77, 60)
  point P1 (12.5, 4)
  dimension "d1" = 25
  dimension "d2" = 64
  dimension "d3" = 4
  dimension "d5" = 8
  dimension "d6" = 5
  dimension "d7" = 5
  dimension "d8" = 5
  dimension "d19" = 12.5
  dimension "d21" = 60
  dimension "d22" = 13.77
  constraint vertical L0
  constraint vertical L1
  constraint coincident L1.end L14.start
  constraint horizontal L2
  constraint perpendicular L2 L3
  constraint parallel L2 L4
  constraint parallel L3 L5
  constraint coincident L6 P0
  constraint coincident L7 P0
  constraint horizontal L8
  constraint perpendicular L8 L9
  constraint parallel L8 L10
  constraint parallel L9 L11
  constraint coincident L12 P1
  constraint coincident L13 P1
  constraint coincident P1 L15.end
  constraint perpendicular L10 L15
  constraint perpendicular L1 L16
  constraint coincident P0 L17.start
  constraint coincident L16 L17.end
  constraint coincident L14 L17.end
  constraint coincident L1 L18.end
  constraint perpendicular L1 L18
  constraint perpendicular L17 L18
  constraint perpendicular L0 L19
  measures "d1" distance of L1.end L0.start
  measures "d2" distance of L1.end L1.start
  measures "d3" distance of L14.end P1
  measures "d5" distance of L3.end L4.end
  measures "d6" distance of L2.end L3.end
  measures "d7" distance of L9.end L10.end
  measures "d8" distance of L8.end L9.end
  measures "d19" distance of L14.end L1.end
  measures "d21" distance of P0 L17.end
  measures "d22" distance of P0 L18.end
extrude "Extrude4" add sketch "Sketch1" along normal blind 1.6 contours L0 L1 L16 L19 | L2 L3 L4 L5 | L8 L9 L10 L11
extrude "Extrude5" add sketch "Sketch1" against normal blind 8.5 contours L2 L3 L4 L5 | L8 L9 L10 L11

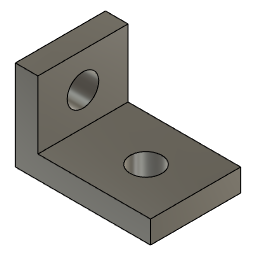
design "Input_Top_Stand"
Autodesk Fusion 360 part; units mm, degrees
sketch "Sketch1" plane through (0, 0, 0) normal (0, 0, 1) x (1, 0, 0)
  line L0 (0, 0) -> (15, 0)
  line L1 (15, 0) -> (15, 10)
  line L2 (15, 10) -> (0, 10)
  line L3 (0, 10) -> (0, 0)
  line L4 (0, 5) -> (9.5, 5)
  circle A0 centre (9.5, 5) radius 1.75
  dimension "d1" = 15
  dimension "d20" = 10
  dimension "d35" = 9.5
  dimension "d36" = 3.5
  constraint horizontal L0
  constraint vertical L1
  constraint coincident L0.start L3.end
  constraint perpendicular L1 L2
  constraint perpendicular L0 L3
  constraint midpoint L3 L4.start
  constraint perpendicular L3 L4
  constraint coincident L4.end A0.centre
  measures "d1" distance of L0.start L0.end
  measures "d20" distance of L0.end L1.end
  measures "d35" distance of L4.start L4.end
  measures "d36" diameter of A0
extrude "Extrude1" add sketch "Sketch1" along normal blind 2.5 contours L0 L1 L2 L3 | A0
extrude "Extrude5" cut sketch "Sketch1" along normal blind 2.5 contours A0
sketch "Sketch5" plane through (0, 0, 0) normal (0, 0, -1) x (1, 0, 0)
  circle A0 centre (9.5, -5) radius 1.75
  line L0 (0, 0) -> (0, -10)
  line L1 (0, -10) -> (15, -10)
  line L2 (15, -10) -> (15, 0)
  line L3 (15, 0) -> (0, 0)
  line L4 (0, 0) -> (2.5, 0)
  line L5 (2.5, 0) -> (2.5, -10)
  line L6 (2.5, -10) -> (0, -10)
  line L7 (0, -10) -> (0, 0)
  dimension "d39" = 2.5
  dimension "d40" = 10
  constraint horizontal L4
  constraint vertical L5
  constraint horizontal L6
  constraint vertical L7
  constraint coincident L0.start L3.end
  measures "d39" distance of L0.start L4.end
  measures "d40" distance of L0.start L0.end
extrude "Extrude6" add sketch "Sketch5" against normal blind 10 contours L0 L1 L3 L4 L5 L6 L7
sketch "Sketch7" plane through (0, 0, 0) normal (-1, 0, 0) x (0, -1, 0)
  line L0 (-10, 0) -> (0, 0)
  line L1 (0, 0) -> (0, 10)
  line L2 (0, 10) -> (-10, 10)
  line L3 (-10, 10) -> (-10, 0)
  line L4 (-5, 0) -> (-5, 6.15)
  circle A0 centre (-5, 6.15) radius 1.75
  dimension "d43" = 6.15
  dimension "d44" = 3.5
  constraint midpoint L0 L4.start
  constraint perpendicular L0 L4
  constraint coincident L4.end A0.centre
  measures "d43" distance of L4.start L4.end
  measures "d44" diameter of A0
extrude "Extrude7" cut sketch "Sketch7" against normal blind 5 contours A0

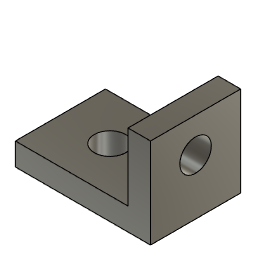
design "Input_Bot_Stand"
Autodesk Fusion 360 part; units mm, degrees
sketch "Sketch1" plane through (0, 0, 0) normal (0, 0, 1) x (1, 0, 0)
  line L0 (0, 0) -> (15, 0)
  line L1 (15, 0) -> (15, 10)
  line L2 (15, 10) -> (0, 10)
  line L3 (0, 10) -> (0, 0)
  line L4 (15, 5) -> (5.5, 5)
  circle A0 centre (5.5, 5) radius 1.75
  dimension "d1" = 15
  dimension "d2" = 10
  dimension "d28" = 9.5
  dimension "d29" = 3.5
  constraint horizontal L0
  constraint vertical L1
  constraint horizontal L2
  constraint vertical L3
  constraint coincident L0.start L3.end
  constraint horizontal L4
  constraint midpoint L1 L4.start
  constraint coincident L4.end A0.centre
  measures "d1" distance of L0.start L0.end
  measures "d2" distance of L0.start L2.end
  measures "d28" distance of L4.start L4.end
  measures "d29" diameter of A0
extrude "Extrude1" add sketch "Sketch1" along normal blind 2.5 contours L0 L1 L2 L3 | A0
extrude "Extrude4" cut sketch "Sketch1" along normal blind 2.5 contours A0
sketch "Sketch5" plane through (0, 0, 0) normal (0, 0, -1) x (1, 0, 0)
  circle A0 centre (5.5, -5) radius 1.75
  line L0 (0, 0) -> (0, -10)
  line L1 (0, -10) -> (15, -10)
  line L2 (15, -10) -> (15, 0)
  line L3 (15, 0) -> (0, 0)
  line L4 (15, -10) -> (12.5, -10)
  line L5 (12.5, -10) -> (12.5, 0)
  line L6 (12.5, 0) -> (15, 0)
  line L7 (15, 0) -> (15, -10)
  dimension "d32" = 2.5
  dimension "d33" = 10
  constraint horizontal L4
  constraint vertical L5
  constraint horizontal L6
  constraint vertical L7
  constraint coincident L1.end L2.start
  measures "d32" distance of L1.end L4.end
  measures "d33" distance of L1.end L2.end
extrude "Extrude5" add sketch "Sketch5" against normal blind 10 contours L1 L2 L3 L4 L5 L6 L7
sketch "Sketch6" plane through (15, 0, 0) normal (1, 0, 0) x (0, 1, 0)
  line L0 (10, 0) -> (10, 10)
  line L1 (10, 10) -> (0, 10)
  line L2 (0, 10) -> (0, 0)
  line L3 (5, 0) -> (5, 6.15)
  circle A0 centre (5, 6.15) radius 1.75
  line L4 (0, 0) -> (10, 0)
  dimension "d36" = 6.15
  dimension "d37" = 3.5
  constraint coincident L3.end A0.centre
  measures "d36" distance of L3.start L3.end
  measures "d37" diameter of A0
extrude "Extrude6" cut sketch "Sketch6" against normal blind 5 contours A0

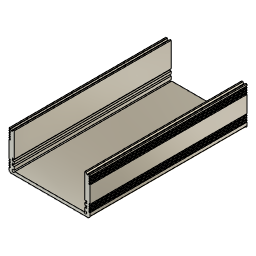
design "Bottom Half"
Autodesk Fusion 360 part; units mm, degrees
sketch "Sketch1" plane through (0, 0, 0) normal (0, 1, 0) x (1, 0, 0)
  line L0 (5, -11) -> (3.2, -11)
  line L1 (74.2, -13) -> (72.4, -13)
  arc A0 (2, 0) -> (0, -2) centre (2, -2) ccw
  line L2 (3.2, -13) -> (5, -13)
  arc A1 (72.4, -4.0966) -> (71.75, -3) centre (73, -3) ccw
  arc A2 (5.4296, -3) -> (5, -3.9431) centre (4.1796, -3) ccw
  line L3 (2, 0) -> (75.4, 0)
  line L4 (3.2, -11) -> (3.2, -13)
  line L5 (74.2, -11) -> (74.2, -13)
  line L6 (72.4, -11) -> (74.2, -11)
  arc A3 (77.4, -2) -> (75.4, 0) centre (75.4, -2) ccw
  line L7 (71.75, -3) -> (5.4296, -3)
  line L8 (72.4, -36.6134) -> (73.6, -36.6134)
  line L9 (77.4, -36.6134) -> (76.2, -36.6134)
  line L10 (74.3, -35.2) -> (75.5, -35.2)
  line L11 (73.6, -36.6134) -> (74.3, -35.2)
  line L12 (75.5, -35.2) -> (76.2, -36.6134)
  line L13 (72.4, -36.6134) -> (73.6, -36.6134)
  line L14 (74.3, -35.2) -> (75.5, -35.2)
  line L15 (73.6, -36.6134) -> (74.3, -35.2)
  line L16 (75.5, -35.2) -> (76.2, -36.6134)
  line L17 (77.4, -36.6134) -> (76.2, -36.6134)
  line L18 (0, -36.6134) -> (1.2, -36.6134)
  line L19 (1.9, -35.2) -> (3.1, -35.2)
  line L20 (1.2, -36.6134) -> (1.9, -35.2)
  line L21 (3.1, -35.2) -> (3.8, -36.6134)
  line L22 (5, -36.6134) -> (3.8, -36.6134)
  line L23 (0, -36.6134) -> (0, -2)
  line L24 (5, -36.6134) -> (5, -13)
  line L25 (77.4, -36.6134) -> (77.4, -2)
  line L26 (72.4, -13) -> (72.4, -36.6134)
  line L27 (5.4296, -3) -> (5.4296, -7) construction
  line L28 (5.4296, -7) -> (5, -7) construction
  line L29 (5, -7) -> (3, -7)
  line L30 (3, -7) -> (3, -8.8)
  line L31 (3, -8.8) -> (5, -8.8)
  line L32 (5, -3.9431) -> (5, -7)
  line L33 (5, -8.8) -> (5, -11)
  line L34 (5, -7) -> (72.4, -7) construction
  line L35 (72.4, -7) -> (74.2, -7)
  line L36 (74.2, -7) -> (74.2, -9)
  line L37 (74.2, -9) -> (72.4, -9)
  line L38 (72.4, -11) -> (72.4, -9)
  line L39 (72.4, -7) -> (72.4, -4.0966)
  dimension "d5" = 2
  dimension "d6" = 2
  dimension "d11" = 1.8
  dimension "d12" = 2
  dimension "d14" = 1.8
  dimension "d15" = 2
  dimension "d19" = 2.5
  dimension "d20" = 2.5
  dimension "d23" = 1.2
  dimension "d24" = 1.2
  dimension "d25" = 1.2
  dimension "d26" = 1.2
  dimension "d27" = 1.2
  dimension "d28" = 1.2
  dimension "d29" = 1.2
  dimension "d30" = 1.2
  dimension "d31" = 1.2
  dimension "d133" = 4
  dimension "d134" = 2
  dimension "d135" = 1.8
  dimension "d136" = 1.8
  dimension "d137" = 2
  constraint horizontal L3
  constraint tangent L3 A3
  constraint coincident origin L3
  constraint tangent A0 L3
  constraint horizontal L7
  constraint vertical L32
  constraint perpendicular L0 L32
  constraint perpendicular L0 L4
  constraint coincident L2.end L32
  constraint perpendicular L2 L32
  constraint perpendicular L5 L6
  constraint collinear L8 L9
  constraint collinear L13 L17
  constraint collinear L18 L22
  constraint tangent A0 L23
  constraint perpendicular L2 L24
  constraint tangent A3 L25
  constraint perpendicular L13 L26
  constraint perpendicular L7 L27
  constraint perpendicular L28 L32
  constraint horizontal L29
  constraint vertical L30
  constraint horizontal L31
  constraint collinear L32 L33
  constraint coincident L34.end L38
  constraint perpendicular L34 L38
  constraint horizontal L35
  constraint vertical L36
  constraint horizontal L37
  constraint collinear L38 L39
  measures "d5" radius of A3
  measures "d6" radius of A0
  measures "d11" distance of L0.end L0.start
  measures "d12" distance of L0.end L2.start
  measures "d14" distance of L5.start L6.start
  measures "d15" distance of L1.start L5.start
  measures "d19" diameter of A1
  measures "d20" diameter of A2
  measures "d23" distance of L8.start L8.end
  measures "d24" distance of L9.start L9.end
  measures "d25" distance of L10.start L10.end
  measures "d26" distance of L8.end L8.start
  measures "d27" distance of L9.start L9.end
  measures "d28" distance of L10.start L10.end
  measures "d29" distance of L18.end L18.start
  measures "d30" distance of L22.start L21.end
  measures "d31" distance of L19.start L19.end
  measures "d133" distance of A2.start L27.end
  measures "d134" distance of L28.end L29.end
  measures "d135" distance of L28.end L31.end
  measures "d136" distance of L34.end L35.end
  measures "d137" distance of L34.end L37.end
extrude "Extrude1" add sketch "Sketch1" along normal blind 150